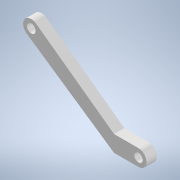
# Autodesk Inventor part: palanca base_proxima
Saved by Autodesk Inventor 2020 (Build 240168000, 168)
## iProperties
Created: 2021-08-20
Part Number: palanca base_proxima
Material: PPS Plastic
Document SubType Name: Modeling
Designer: chalo
Density: 1.637 g/cm^3
Appearance: Smooth - White
Author: chalo
Autodesk Inventor part; units mm, degrees
ref_plane "YZ Plane" through (0, 0, 0) normal (1, 0, 0) x (0, 1, 0)
ref_plane "XZ Plane" through (0, 0, 0) normal (0, 1, 0) x (-1, 0, 0)
ref_plane "XY Plane" through (0, 0, 0) normal (0, 0, 1) x (1, 0, 0)
sketch "Sketch1" plane through (0, 0, 0) normal (0, 0, 1) x (1, 0, 0)
  circle A0 centre (-25.35, -26.8891) radius 1.55 projected
  circle A1 centre (-25.35, -26.8891) radius 3
  circle A2 centre (-64.85, -5.4402) radius 1.6 projected
  circle A3 centre (-64.85, -5.4402) radius 3
  line L0 (-26.7816, -29.5255) -> (-66.2816, -8.0766) construction
  line L1 (-23.9184, -24.2527) -> (-63.4184, -2.8038) construction
  line L2 (-23.9184, -24.2527) -> (-31.4868, -20.143)
  line L3 (-26.7816, -29.5255) -> (-34.35, -25.4158)
  line L4 (-31.4868, -20.143) -> (-38.5358, -8.639)
  line L5 (-34.35, -25.4158) -> (-41.399, -13.9118)
  line L6 (-41.399, -13.9118) -> (-59.85, -13.9118)
  line L7 (-38.5358, -8.639) -> (-56.9868, -8.639)
  line L8 (-56.9868, -8.639) -> (-62.8104, -3.2402)
  line L9 (-32.35, -16.7754) -> (-65.35, -16.7754)
  line L10 (-32.35, -5.7754) -> (-57.816, -5.7754)
  line L11 (-32.35, -5.7754) -> (-32.35, -16.7754) construction
  line L12 (-32.35, -11.2754) -> (-52.35, -11.2754) construction
  line L13 (-56.9868, -8.639) -> (-56.9868, -13.9118) construction
  line L14 (-63.35, -12.7754) -> (-63.35, -16.4711) construction
  line L15 (-59.85, -13.9118) -> (-66.2816, -8.0766)
  point P0 (0, 0)
  point P1 (-56.9868, -11.2754)
  dimension "d0" = 6
  dimension "d1" = 6
  dimension "d5" = 30
  dimension "d6" = 30
  dimension "d7" = 6
  dimension "d8" = 6
  dimension "d9" = 6
  dimension "d10" = 9
  dimension "d11" = 20
  dimension "d12" = 3.5
  constraints: 30 end point, 5 point on circle, 5 tangent, 4 horizontal, 3 point on line, 2 centre point, 2 coincident, 2 midpoint, 2 vertical, 1 horizontal alignment, 1 parallel, 4 other
  measures "d0" diameter of A1
  measures "d1" diameter of A3
  measures "d5" angle of L0 L5
  measures "d6" angle of L1 L4
  measures "d7" distance of L2.end L3.end
  measures "d8" distance of L7.end L6.end
  measures "d9" distance of L4.end L5.end
  measures "d10" horizontal distance of A0.centre L3.end
  measures "d11" distance of L12.start L12.end
  measures "d12" distance from line of L14 L6.end
extrude "Extrusion1" add sketch "Sketch1" along normal mid plane 3.8
chamfer "Chamfer1" distance 2 angle 45 3 edges at (-59.85, -13.9118, 0) (-38.5358, -8.639, 0) (-34.35, -25.4158, 0)
body "Solid1"
